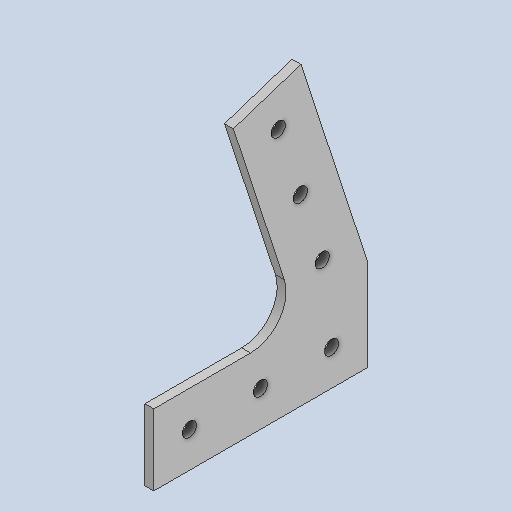
# Autodesk Inventor part: Bot_ang_gus
Saved by Autodesk Inventor 2024 (Build 280153000, 153)
## iProperties
Created: 2023-04-21
Part Number: Bot_ang_gus
Material: Generic
Document SubType Name: Modeling
Designer: legom
Density: 1 g/cm^3
Appearance: Default
Author: legom
Autodesk Inventor part; units mm, degrees
ref_plane "YZ Plane" through (0, 0, 0) normal (1, 0, 0) x (0, 1, 0)
ref_plane "XZ Plane" through (0, 0, 0) normal (0, 1, 0) x (-1, 0, 0)
ref_plane "XY Plane" through (0, 0, 0) normal (0, 0, 1) x (1, 0, 0)
sketch "Sketch1" plane through (0, 0, 0) normal (1, 0, 0) x (0, 1, 0)
  line L0 (0, 0) -> (25.4, 0)
  line L1 (25.4, 0) -> (25.4, 76.2)
  line L2 (25.4, 76.2) -> (0, 76.2)
  line L3 (0, 76.2) -> (0, 0)
  line L4 (25.4, 0) -> (33.274, 0)
  line L5 (33.274, 0) -> (105.7201, 23.622)
  line L6 (105.7201, 23.622) -> (97.8461, 47.7707)
  line L7 (97.8461, 47.7707) -> (25.4, 24.1487)
  circle A0 centre (41.4114, 16.0114) radius 2.5527
  circle A1 centre (12.7, 12.7) radius 2.5527
  line L8 (25.4, 24.1487) -> (33.274, 0)
  circle A2 centre (12.7, 38.1) radius 2.5527
  circle A3 centre (12.7, 63.5) radius 2.5527
  circle A4 centre (65.5601, 23.8854) radius 2.5527
  circle A5 centre (89.7088, 31.7594) radius 2.5527
  point P0 (12.7, 0)
  dimension "d0" = 25.4
  dimension "d1" = 76.2
  dimension "d2" = 7.874
  dimension "d3" = 76.2
  dimension "d4" = 25.4
  dimension "d5" = 5.1054
  dimension "d6" = 5.1054
  dimension "d7" = 12.7
  dimension "d8" = 12.7
  dimension "d9" = 12.7
  dimension "d10" = 12.7
  dimension "d20" = 25.4
  dimension "d27" = 25.4
  constraints: 18 end point, 6 centre point, 3 parallel, 3 perpendicular, 2 horizontal, 1 midpoint, 1 point on line, 1 vertical, 9 other
  measures "d0" distance of L2.end L1.end
  measures "d1" distance of L1.end L0.end
  measures "d2" distance of L0.end L4.end
  measures "d3" distance of L4.end L5.end
  measures "d4" distance between parallel lines of L5 L7
  measures "d5" diameter of A0
  measures "d6" diameter of A1
  measures "d7" distance of point (12.7, 0) A1.centre
  measures "d8" distance from line of A1.centre L3
  measures "d9" distance from line of L7 A0.centre
  measures "d10" distance from line of L8 A0.centre
  measures "d20" distance of A1.centre A2.centre
  measures "d27" distance of A0.centre A4.centre
extrude "Extrusion1" add sketch "Sketch1" along normal blind 3.175
fillet "Fillet1" radius 12.7 1 edges at (1.5875, 25.4, 24.1487)
body "Solid1"
